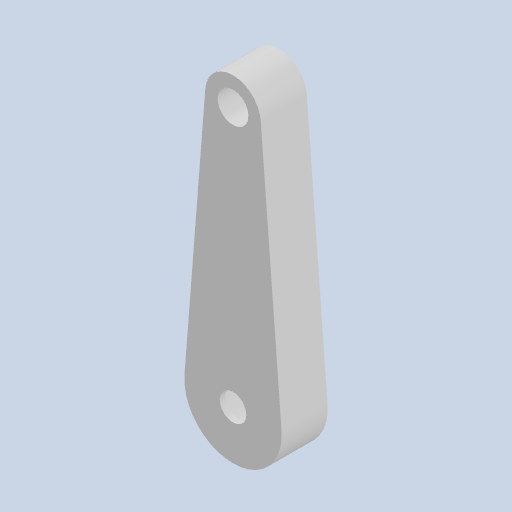
# Autodesk Inventor part: shatun_main
Saved by Autodesk Inventor 2022 (Build 260153000, 153)
## iProperties
Created: 2024-10-19
Part Number: shatun_main
Material: Типовые
Document SubType Name: Modeling
Designer: Andrey
Density: 1 g/cm^3
Appearance: По умолчанию
Author: Andrey
Autodesk Inventor part; units mm, degrees
ref_plane "YZ Plane" through (0, 0, 0) normal (1, 0, 0) x (0, 1, 0)
ref_plane "XZ Plane" through (0, 0, 0) normal (0, 1, 0) x (-1, 0, 0)
ref_plane "XY Plane" through (0, 0, 0) normal (0, 0, 1) x (1, 0, 0)
sketch "Эскиз1" plane through (0, 0, 0) normal (0, 0, 1) x (1, 0, 0)
  circle A0 centre (0, 0) radius 1.925 projected
  circle A1 centre (0, 0) radius 1.9
  circle A2 centre (0, 0) radius 3.5
  circle A3 centre (0, 0) radius 18.645 projected
  line L0 (0, 69.6007) -> (0, -10.6967) projected
  circle A4 centre (0, 18.645) radius 1.1
  circle A5 centre (0, 18.645) radius 2
  line L1 (-1.9935, 18.8059) -> (-3.4887, 0.2816)
  line L2 (3.4887, 0.2816) -> (1.9935, 18.8059)
  point P0 (0, 0)
  point P1 (2.0153, 18.5358)
  point P2 (1.9971, 18.5377)
  point P3 (-1.9971, 18.5377)
  point P4 (-2.0153, 18.5358)
  dimension "d0" = 3.8
  dimension "d1" = 7
  dimension "d2" = 2.2
  dimension "d3" = 4
  constraints: 4 centre point, 4 end point, 4 point on circle, 4 tangent, 3 coincident, 1 point on line, 2 other
  measures "d0" diameter of A1
  measures "d1" diameter of A2
  measures "d2" diameter of A4
  measures "d3" diameter of A5
extrude "Выдавливание1" add sketch "Эскиз1" along normal mid plane 2.9 contours A0 L0 A2 | A0 L0 A2 | L0 A5 A3 L2 A2 | A2 L1 A3 A5 L0 | A5 A3 A4 L0 | L0 A4 A3 A5 | A3 A5 L2 | L1 A5 A3 | A5 L0 A4 A3 | A3 A4 L0 A5
sketch "Эскиз2" plane through (0, 0, 1.45) normal (0, 0, 1) x (1, 0, 0)
  line L0 (3.4887, 0.2816) -> (1.9935, 18.8059) projected
  arc A0 (1.9935, 18.8059) -> (-1.9935, 18.8059) centre (0, 18.645) ccw projected
  line L1 (-1.9935, 18.8059) -> (-3.4887, 0.2816) projected
  arc A1 (-3.4887, 0.2816) -> (3.4887, 0.2816) centre (0, 0) ccw projected
  circle A2 centre (0, 0) radius 1.925 projected
  circle A3 centre (0, 18.645) radius 1.1 projected
  circle A4 centre (0, 0) radius 0.95
  point P0 (0, 0)
  dimension "d8" = 1.9
  constraints: 1 centre point, 1 coincident
  measures "d8" diameter of A4
extrude "Выдавливание2" add sketch "Эскиз2" along normal blind 0.4 contours A1 L1 A0 L0 | A2
